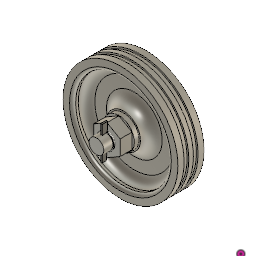
QWEQ (4) (Autodesk Fusion 360 design; units mm, degrees)
Autodesk Fusion 360 part; units mm, degrees
sketch "Sketch1" plane through (0, 0, 0) normal (1, 0, 0) x (0, 1, 0) in component "Piston"
  line L0 (50, 0) -> (190, 0)
  line L1 (175, 45) -> (85, 36)
  line L2 (175, 45) -> (175, 223)
  line L3 (175, 223) -> (151, 223)
  line L4 (151, 223) -> (151, 205)
  line L5 (151, 205) -> (133, 205)
  line L6 (133, 205) -> (133, 223)
  line L7 (133, 223) -> (115, 223)
  line L8 (115, 223) -> (115, 205)
  line L9 (115, 205) -> (97, 205)
  line L10 (97, 205) -> (97, 223)
  line L11 (97, 223) -> (73, 223)
  line L12 (73, 223) -> (73, 185)
  line L13 (85, 36) -> (85, 66)
  arc A0 (85, 66) -> (127, 108) centre (85, 108) ccw
  line L14 (127, 108) -> (127, 153)
  line L15 (73, 185) -> (95, 185)
  arc A1 (127, 153) -> (95, 185) centre (95, 153) ccw
  dimension "d10" = 38
  dimension "d14" = 32
  constraint horizontal L0
  constraint vertical L2
  constraint perpendicular L2 L3
  constraint perpendicular L3 L4
  constraint perpendicular L4 L5
  constraint perpendicular L5 L6
  constraint perpendicular L6 L7
  constraint perpendicular L5 L8
  constraint perpendicular L8 L9
  constraint perpendicular L7 L10
  constraint perpendicular L10 L11
  constraint perpendicular L11 L12
  constraint vertical L13
  constraint tangent A0 L14
  constraint vertical L14
  constraint perpendicular L14 L15
  constraint tangent L14 A1
  constraint tangent L15 A1
  measures "d10" distance of L11.end L12.end
  measures "d14" radius of A1
revolve "Revolve1" add sketch "Sketch1" angle 360 about axis through (0, 50, 0) along (0, 1, 0) makes body 1 in component "Piston"
fillet "Fillet1" radius 12 1 edges at (-172.4806, 73, 66.8989) on bodies 1 in component "Piston"
move_body "Move1" bodies 1 to x (1, 0, 0) y (0, 1, 0) z (0, 0, 1) at (0, 450, 0) in component "Piston"
sketch "Sketch1 (2)" plane through (0, 0, 0) normal (1, 0, 0) x (0, 1, 0) in component "Piston Rod"
  line L0 (350, 0) -> (350, 42)
  line L1 (350, 42) -> (300, 42)
  line L2 (300, 42) -> (300, 45)
  line L3 (300, 45) -> (210, 36)
  line L4 (210, 36) -> (210, 33)
  line L5 (210, 33) -> (141, 33)
  line L6 (141, 33) -> (141, 28.4758)
  line L7 (141, 28.4758) -> (105, 28.4758)
  line L8 (105, 28.4758) -> (105, 0)
  line L9 (105, 0) -> (350, 0)
  line L10 (360, 0) -> (90, 0)
  dimension "d22" = 36
  constraint vertical L0
  constraint perpendicular L0 L1
  constraint perpendicular L1 L2
  constraint perpendicular L4 L5
  constraint perpendicular L5 L6
  constraint perpendicular L6 L7
  constraint perpendicular L7 L8
  constraint perpendicular L0 L9
  constraint perpendicular L8 L10
  measures "d22" distance of L6.end L7.end
revolve "Revolve1'" add sketch "Sketch1 (2)" angle 360 about axis through (0, 360, 0) along (0, -1, 0) separate body makes body 2 in component "Piston Rod"
thread "Thread1" "ISO Metric profile 65.0 M65x4 6g" major diameter 64.7025 minor diameter 60.1258 pitch 4 angle 60 resizes the face on face at (1.6449, 187, 32.959) on bodies 2 in component "Piston Rod"
move_body "Move1'" bodies 2 to x (1, 0, 0) y (0, 1, 0) z (0, 0, 1) at (0, 0, -32.5) in component "Piston Rod"
sketch "Sketch2" plane through (0, 0, 0) normal (0, 0, 1) x (1, 0, 0) in component "Piston Rod"
  line L0 (3, 141) -> (3, 144)
  line L1 (3, 144) -> (-3, 144)
  line L2 (-3, 144) -> (-3, 126)
  line L3 (-3, 144) -> (15, 144) construction
  line L4 (-3, 126) -> (3, 126)
  line L5 (3, 126) -> (3, 141)
  point P0 (0, 141)
  dimension "d24" = 3
  dimension "d25" = 90
  dimension "d26" = 6
  dimension "d27" = 90
  dimension "d28" = 18
  constraint horizontal L3
  constraint perpendicular L0 L4
  measures "d24" distance of P0 L0.start
  measures "d25" angle of L0 L1
  measures "d26" distance of L0.end L1.end
  measures "d27" angle of L2 L3
  measures "d28" distance of L1.end L2.end
extrude "Extrude1" cut sketch "Sketch2" against normal blind 66 bodies 2 in component "Piston Rod"
sketch "Sketch1 (3)" plane through (0, 0, 0) normal (0, 0, 1) x (1, 0, 0) in component "Piston Ring"
  circle A0 centre (0, -500) radius 198
  circle A1 centre (0, -500) radius 216.5
  dimension "d31" = 396
  dimension "d32" = 433
  constraint concentric A0 A1
  measures "d31" diameter of A0
  measures "d32" diameter of A1
extrude "Extrude1'" add sketch "Sketch1 (3)" along normal blind 18 separate body makes body 3 in component "Piston Ring"
sketch "Sketch2 (2)" plane through (0, 0, 0) normal (0, 1, 0) x (1, 0, 0) in component "Piston Ring"
move_body "Move1''" bodies 3 to x (1, 0, 0) y (0, 1, 0) z (0, 0, 1) at (-325, 500, 0) in component "Piston Ring"
move_body "Move2" bodies 3 to x (1, 0, 0) y (0, 1, 0) z (0, 0, 1) at (-100, 216.5, 0) in component "Piston Ring"
sketch "Sketch3" plane through (0, 0, 0) normal (0, 1, 0) x (1, 0, 0) in component "Piston Ring"
  line L0 (-641.5, 0) -> (-208.5, 0)
  line L1 (-227, -18) -> (-623, -18)
  line L2 (-425, 0) -> (-415.1892, -18)
  line L3 (-415.1892, -18) -> (-407.1892, -18)
  line L4 (-425, 0) -> (-417, 0)
  line L5 (-407.1892, -18) -> (-417, 0)
  dimension "d37" = 8
  dimension "d38" = 8
  constraint midpoint L0 L2.start
  constraint coincident L1 L2.end
  constraint horizontal L3
  constraint horizontal L4
  measures "d37" distance of L2.end L3.end
  measures "d38" distance of L2.start L4.end
extrude "Extrude2" add sketch "Sketch3" against normal blind 18 separate body makes body 4 in component "Piston Ring"
extrude "Extrude3" cut 1 faces at (-419.0631, -18, 6) along direction (0, 1, 0) blind 38 on bodies 4 bodies 3 4 in component "Piston Ring"
copy_body "CopyPasteBodies1" bodies 3 makes body 5 in component "Piston Ring"
move_body "Move3" bodies 5 to x (1, 0, 0) y (0, 1, 0) z (0, 0, 1) at (-500, 0, 0) in component "Piston Ring"
copy_body "Body->Comp1" bodies 5 removing the originals makes body 6 in component "Component"
sketch "Sketch1 (4)" plane through (0, 0, 0) normal (1, 0, 0) x (0, 1, 0) in component "Cotter"
  line L0 (565, -205) -> (565, 205)
  line L1 (850, 0) -> (850, 130)
  line L2 (850, 130) -> (871, 130)
  line L3 (850, 0) -> (866.67, 0)
  line L4 (871, 130) -> (866.67, 0)
  constraint vertical L1
  constraint horizontal L2
  constraint horizontal L3
extrude "Extrude1''" add sketch "Sketch1 (4)" along normal blind 6 separate body makes body 7 in component "Cotter"
sketch "Sketch1 (5)" plane through (0, 0, 0) normal (1, 0, 0) x (0, 1, 0) in component "Piston Nut"
  circle A0 centre (1125, 0) radius 60
  dimension "d48" = 120
  measures "d48" diameter of A0
extrude "Extrude1'''" add sketch "Sketch1 (5)" along normal blind 18 separate body makes body 8 in component "Piston Nut"
sketch "Sketch2 (3)" plane through (18, 0, 0) normal (1, 0, 0) x (0, 1, 0) in component "Piston Nut"
  circle A0 centre (1125, 0) radius 60
  line L0 (1176, 29.4449) -> (1125, 58.8897)
  line L1 (1125, 58.8897) -> (1074, 29.4449)
  line L2 (1074, 29.4449) -> (1074, -29.4449)
  line L3 (1074, -29.4449) -> (1125, -58.8897)
  line L4 (1125, -58.8897) -> (1176, -29.4449)
  line L5 (1176, -29.4449) -> (1176, 29.4449)
  point P0 (1125, 0)
  dimension "d51" = 51
  constraint coincident P0 A0.centre
  measures "d51" distance of P0 L5
extrude "Extrude2'" add sketch "Sketch2 (3)" along normal blind 48 contours L0 L1 L2 L3 L4 L5 bodies 8 in component "Piston Nut"
sketch "Sketch3 (2)" plane through (66, 0, 0) normal (1, 0, 0) x (0, 1, 0) in component "Piston Nut"
  line L0 (1176, -29.4449) -> (1176, 29.4449)
  line L1 (1176, 29.4449) -> (1125, 58.8897)
  line L2 (1125, 58.8897) -> (1074, 29.4449)
  line L3 (1074, 29.4449) -> (1074, -29.4449)
  line L4 (1074, -29.4449) -> (1125, -58.8897)
  line L5 (1125, -58.8897) -> (1176, -29.4449)
  line L6 (1176, -29.4449) -> (1172.3228, -23.0758)
  circle A0 centre (1125, 0) radius 33
  dimension "d54" = 66
  constraint coincident L0.start L5.end
  constraint perpendicular L5 L6
  measures "d54" diameter of A0
extrude "Extrude3'" cut sketch "Sketch3 (2)" against normal blind 66 contours A0 bodies 8 in component "Piston Nut"
thread "Thread1'" "ISO Metric profile 65.0 M65x4 6H" major diameter 65.4462 minor diameter 60.9699 pitch 4 angle 60 resizes the face on face at (22, 1130.7304, 32.4987) on bodies 8 in component "Piston Nut"
extrude "Extrude4" cut 1 faces at (66, 1169.1617, 0) along direction (-1, 0, 0) blind 2 on bodies 8 bodies 8 in component "Piston Nut"
copy_body "Body->Comp1'" bodies 2 removing the originals makes body 9 in component "Piston Rod (1)"
copy_body "Body->Comp2" bodies 3 removing the originals makes body 10 in component "Piston Ring (1)"
copy_body "Body->Comp3" bodies 4 removing the originals in component "Piston Ring 2"
copy_body "Body->Comp1''" bodies 7 removing the originals makes body 11 in component "Cotter (1)"
copy_body "Body->Comp1'''" bodies 8 removing the originals makes body 12 in component "Piston Nut (1)"
copy_body "Body->Comp1''''" bodies 1 removing the originals makes body 13 in component "Piston (1)"
component "Piston" placed x (1, 0, 0) y (0, 1, 0) z (0, 0, 1) at (0, 0, 0)
component "Piston Rod" placed x (1, 0, 0) y (0, 1, 0) z (0, 0, 1) at (0, 325, 32.5) in component "Piston"
component "Piston (1)" placed x (1, 0, 0) y (0, 1, 0) z (0, 0, 1) at (0, 0, 0) in component "Piston"
component "Piston Ring" placed x (1, 0, 0) y (0, 0, 1) z (0, -1, 0) at (425, 240, -249) in component "Piston Rod"
component "Piston Rod (1)" placed x (1, 0, 0) y (0, 1, 0) z (0, 0, 1) at (0, 0, 0) in component "Piston Rod"
component "Component" placed x (1, 0, 0) y (0, 1, 0) z (0, 0, 1) at (500, 0, -36) in component "Piston Ring"
component "Cotter" placed x (1, 0, 0) y (0, 0, -1) z (0, 1, 0) at (-428, 151.5, 965.5) in component "Piston Ring"
component "Piston Ring (1)" placed x (1, 0, 0) y (0, 1, 0) z (0, 0, 1) at (0, 0, 0) in component "Piston Ring"
component "Piston Ring 2" placed x (1, 0, 0) y (0, 1, 0) z (0, 0, 1) at (0, 0, 0) in component "Piston Ring"
component "Piston Nut" placed x (0, -1, 0) y (1, 0, 0) z (0, 0, 1) at (-1122, 935.5, 65) in component "Cotter"
component "Cotter (1)" placed x (1, 0, 0) y (0, 1, 0) z (0, 0, 1) at (0, 0, 0) in component "Cotter"
component "Piston Nut (1)" placed x (1, 0, 0) y (0, 1, 0) z (0, 0, 1) at (0, 0, 0) in component "Piston Nut"
